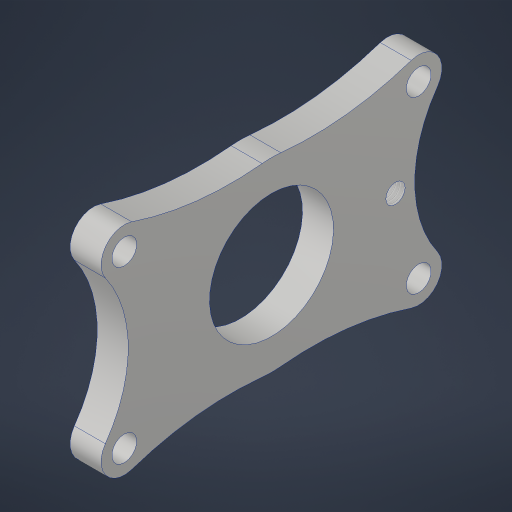
# Autodesk Inventor part: AR-021
Saved by Autodesk Inventor 2023.4 (Build 274418000, 418)
## iProperties
Created: 2025-02-28
Part Number: AR-021
Material: Aluminum 6061
Document SubType Name: Modeling
Designer: slick
Density: 2.7 g/cm^3
Appearance: Aluminum - Flat
Author: slick
Autodesk Inventor part; units mm, degrees
ref_plane "YZ Plane" through (0, 0, 0) normal (1, 0, 0) x (0, 1, 0)
ref_plane "XZ Plane" through (0, 0, 0) normal (0, 1, 0) x (-1, 0, 0)
ref_plane "XY Plane" through (0, 0, 0) normal (0, 0, 1) x (1, 0, 0)
sketch "Sketch1" plane through (0, 0, 0) normal (1, 0, 0) x (0, 1, 0)
  line L0 (-17.4625, -30.1625) -> (17.4625, -30.1625) construction
  line L1 (17.4625, -30.1625) -> (17.4625, 30.1625) construction
  line L2 (17.4625, 30.1625) -> (-17.4625, 30.1625) construction
  line L3 (-17.4625, 30.1625) -> (-17.4625, -30.1625) construction
  line L4 (-17.4625, -30.1625) -> (17.4625, 30.1625) construction
  line L5 (17.4625, -30.1625) -> (-17.4625, 30.1625) construction
  circle A0 centre (17.4625, 30.1625) radius 4.7625 construction
  circle A1 centre (-17.4625, 30.1625) radius 4.7625 construction
  circle A2 centre (-17.4625, -30.1625) radius 4.7625 construction
  circle A3 centre (17.4625, -30.1625) radius 4.7625 construction
  circle A4 centre (0, 0) radius 12.7
  circle A5 centre (0, 0) radius 19.05 construction
  arc A6 (21.9743, 28.6376) -> (18.9533, 1.9166) centre (82.1311, 8.3053) ccw
  arc A7 (18.9533, -1.9166) -> (21.9743, -28.6376) centre (82.1311, -8.3053) ccw
  arc A8 (14.7053, -34.0457) -> (-14.7053, -34.0457) centre (0, -54.7559) ccw
  arc A9 (-21.9743, -28.6376) -> (-18.9533, -1.9166) centre (-82.1311, -8.3053) ccw
  arc A10 (-18.9533, 1.9166) -> (-21.9743, 28.6376) centre (-82.1311, 8.3053) ccw
  arc A11 (-14.7053, 34.0457) -> (14.7053, 34.0457) centre (0, 54.7559) ccw
  arc A12 (21.9743, 28.6376) -> (14.7053, 34.0457) centre (17.4625, 30.1625) ccw
  arc A13 (14.7053, -34.0457) -> (21.9743, -28.6376) centre (17.4625, -30.1625) ccw
  arc A14 (-21.9743, -28.6376) -> (-14.7053, -34.0457) centre (-17.4625, -30.1625) ccw
  arc A15 (-14.7053, 34.0457) -> (-21.9743, 28.6376) centre (-17.4625, 30.1625) ccw
  arc A16 (-18.9533, 1.9166) -> (-18.9533, -1.9166) centre (0, 0) ccw
  arc A17 (18.9533, -1.9166) -> (18.9533, 1.9166) centre (0, 0) ccw
  point P0 (0, 0)
  point P1 (0, 0)
  point P2 (0, -25.4)
  point P3 (14.7053, -34.0457)
  dimension "d1" = 34.925
  dimension "d2" = 60.325
  dimension "d3" = 25.4
  dimension "d4" = 9.525
  dimension "d5" = 25.4
  dimension "d6" = 6.35
  dimension "d7" = 63.5
  dimension "d8" = 25.4
  constraints: 37 point on circle, 18 centre point, 16 coincident, 12 end point, 12 tangent, 8 equal radius, 2 midpoint, 2 parallel, 1 horizontal, 1 perpendicular, 1 vertical alignment
  measures "d1" distance of L0.start L0.end
  measures "d2" distance of L0.end L1.end
  measures "d3" distance of point (0, -25.4) point (0, 0)
  measures "d4" diameter of A0
  measures "d5" diameter of A4
  measures "d6" radial gap between concentric circles of A4 A5
  measures "d7" radius of A6
  measures "d8" radius of A11
extrude "Extrusion1" add sketch "Sketch1" along normal blind 6.35
hole "Hole1" at (0, 17.4625, 30.1625) at (0, 17.4625, -30.1625) at (0, -17.4625, -30.1625) at (0, -17.4625, 30.1625) direction (1, 0, 0) diameter 5.1054 end through all clearance for "Flat Head Machine Screw (82)" size "#10" standard "Ansi Unified Screw Threads"
hole "Hole2" at (0, 0, -25.4) direction (1, 0, 0) diameter 3.9624 end through all thread size "10-32 UNF" class "2B" standard "ANSI Unified Screw Threads"
body "Solid1"
